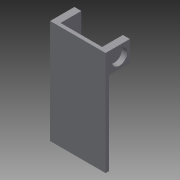
# Autodesk Inventor part: BassGtrBotBase
Saved by Autodesk Inventor 2015 (Build 190159000, 159)
## iProperties
Created: 2016-04-21
Part Number: BassGtrBotBase
Material: Generic
Document SubType Name: Modeling
Designer: Hatch
Density: 1 g/cm^3
Appearance: Default
Author: Hatch
Autodesk Inventor part; units mm, degrees
ref_plane "YZ Plane" through (0, 0, 0) normal (1, 0, 0) x (0, 1, 0)
ref_plane "XZ Plane" through (0, 0, 0) normal (0, 1, 0) x (-1, 0, 0)
ref_plane "XY Plane" through (0, 0, 0) normal (0, 0, 1) x (1, 0, 0)
sketch "Sketch1" plane through (0, 0, 0) normal (0, 1, 0) x (-1, 0, 0)
  line L0 (-40, 50) -> (40, 50)
  line L1 (40, 50) -> (40, -50)
  line L2 (40, -50) -> (-40, -50)
  line L3 (-40, -50) -> (-40, 50)
  line L4 (-40, 50) -> (40, -50) construction
  line L5 (40, 50) -> (-40, -50) construction
  point P0 (0, 0)
  dimension "d0" = 80
  dimension "d1" = 100
  constraints: 12 end point, 2 midpoint, 2 parallel, 1 horizontal, 1 perpendicular
  measures "d0" distance of L1.end L2.end
  measures "d1" distance of L0.end L1.end
extrude "Extrusion1" add sketch "Sketch1" along normal blind 5
sketch "Sketch2" plane through (0, 5, 0) normal (0, 1, 0) x (1, 0, 0)
  line L0 (-40, -50) -> (-30, -50)
  line L1 (-30, -50) -> (-30, -20)
  line L2 (-30, -20) -> (-40, -20)
  line L3 (-40, -20) -> (-40, -50)
  line L4 (40, -50) -> (30, -50)
  line L5 (30, -50) -> (30, -20)
  line L6 (30, -20) -> (40, -20)
  line L7 (40, -20) -> (40, -50)
  point P0 (0, 0)
  dimension "d4" = 10
  dimension "d5" = 30
  dimension "d6" = 10
  dimension "d7" = 30
  constraints: 16 end point, 4 parallel, 2 horizontal, 2 perpendicular
  measures "d4" distance of L2.end L1.end
  measures "d5" distance of L1.end L0.end
  measures "d6" distance of L5.end L6.end
  measures "d7" distance of L4.end L5.end
extrude "Extrusion2" add sketch "Sketch2" along normal blind 30
sketch "Sketch3" plane through (-40, 0, -50) normal (-1, 0, 0) x (0, 0, 1)
  circle A0 centre (85, 20) radius 11
  point P0 (50, 0)
  dimension "d10" = 22
  constraints: 1 centre point
  measures "d10" diameter of A0
extrude "Extrusion3" cut sketch "Sketch3" against normal blind 7.5
sketch "Sketch4" plane through (40, 0, 50) normal (1, 0, 0) x (0, 0, -1)
  circle A0 centre (15, 20) radius 11 projected
  circle A1 centre (15, 20) radius 11
  point P0 (50, 0)
  constraints: 1 centre point, 1 coincident
extrude "Extrusion4" cut sketch "Sketch4" against normal blind 7.5
sketch "Sketch6" plane through (40, 0, -50) normal (0, 0, -1) x (-1, 0, 0)
  line L0 (80, 5) -> (0, 5)
  line L1 (0, 5) -> (0, 0)
  line L2 (0, 0) -> (80, 0)
  line L3 (80, 0) -> (80, 5)
  point P0 (40, 0)
  constraints: 8 end point, 2 parallel, 1 horizontal, 1 perpendicular
extrude "Extrusion5" add sketch "Sketch6" along normal blind 50
body "Solid1"
